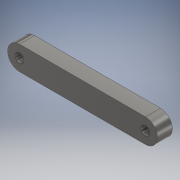
# Autodesk Inventor part: biellette2
Saved by Autodesk Inventor 2017 SP1 (Build 210196100, 196)
## iProperties
Part Number: biellette2
Material: Acier inoxydable
Document SubType Name: Modeling
Designer: Biscuit
Density: 8 g/cm^3
Appearance: Semi-poli
Author: Biscuit
Autodesk Inventor part; units mm, degrees
ref_plane "YZ Plane" through (0, 0, 0) normal (1, 0, 0) x (0, 1, 0)
ref_plane "XZ Plane" through (0, 0, 0) normal (0, 1, 0) x (-1, 0, 0)
ref_plane "XY Plane" through (0, 0, 0) normal (0, 0, 1) x (1, 0, 0)
sketch "Esquisse1" plane through (0, 0, 0) normal (0, 1, 0) x (-1, 0, 0)
  line L0 (0, 0) -> (50, 0)
  line L1 (50, 0) -> (50, -8)
  line L2 (50, -8) -> (0, -8)
  line L3 (0, -8) -> (0, 0)
  circle A0 centre (46, -4) radius 1.5
  circle A1 centre (4, -4) radius 1.5
  dimension "d0" = 8
  dimension "d1" = 50
  dimension "d2" = 3
  dimension "d3" = 3
  dimension "d4" = 4
  dimension "d5" = 4
  dimension "d6" = 4
  dimension "d7" = 4
  constraints: 8 end point, 2 centre point, 2 parallel, 1 horizontal, 1 perpendicular
  measures "d0" distance of L0.end L1.end
  measures "d1" distance of L1.end L2.end
  measures "d2" diameter of A0
  measures "d3" diameter of A1
  measures "d4" distance from line of L2 A0.centre
  measures "d5" distance from line of L1 A0.centre
  measures "d6" distance from line of L2 A1.centre
  measures "d7" distance from line of L3 A1.centre
extrude "Extrusion1" add sketch "Esquisse1" along normal blind 5
fillet "Congé1" radius 4 4 edges at (-50, 2.5, 0) (-50, 2.5, -8) (0, 2.5, 0) (0, 2.5, -8)
equation "\"d3\" = d2"
equation "\"d4\" = 0.5 * d0"
equation "\"d5\" = d4"
equation "\"d6\" = d4"
equation "\"d7\" = d5"
